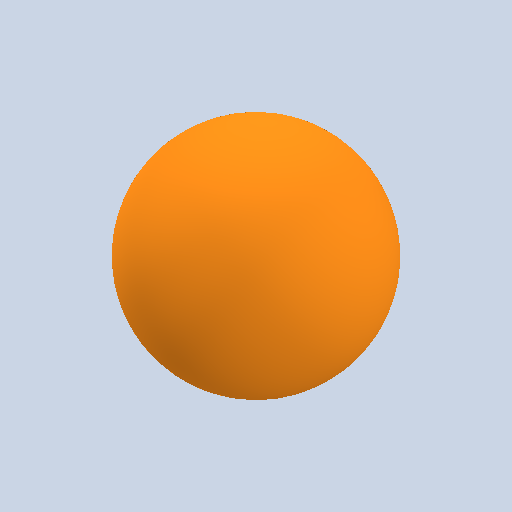
# Autodesk Inventor part: バスケボール（仮）
Saved by Autodesk Inventor 2025.1 (Build 291241000, 241)
## iProperties
Created: 2024-10-06
Part Number: バスケボール（仮）
Material: PAEK 樹脂
Document SubType Name: Modeling
Designer: ryogo
Density: 1.32 g/cm^3
Appearance: オレンジ
Mass: 10164.1 g
Surface Area: 1885.74 cm^2
Volume: 7700.11 cm^3
Author: ryogo
Autodesk Inventor part; units mm, degrees
ref_plane "YZ Plane" through (0, 0, 0) normal (1, 0, 0) x (0, 1, 0)
ref_plane "XZ Plane" through (0, 0, 0) normal (0, 1, 0) x (-1, 0, 0)
ref_plane "XY Plane" through (0, 0, 0) normal (0, 0, 1) x (1, 0, 0)
sketch "スケッチ1" plane through (0, 0, 0) normal (0, 1, 0) x (-1, 0, 0)
  circle A0 centre (0, 0) radius 122.5
  line L0 (122.5, 0) -> (-122.5, 0)
  dimension "d0" = 245
  constraints: 2 end point, 2 point on circle, 1 centre point, 1 coincident, 1 horizontal
  measures "d0" diameter of A0
revolve "回転1" add sketch "スケッチ1" angle 360 about axis through (-122.5, 0, 0) along (1, 0, 0) picked at (21.8796, -54.7864) contours A0 L0
